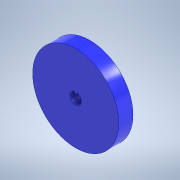
# Autodesk Inventor part: celestronMountDecHandle
Saved by Autodesk Inventor 2021.1 (Build 251245000, 245)
## iProperties
Created: 2020-07-29
Part Number: celestronMountDecHandle
Material: PC/ABS Plastic
Document SubType Name: Modeling
Designer: robst
Density: 0.357273 g/cm^3
Appearance: Blue - Wall Paint - Glossy
Author: robst
Autodesk Inventor part; units mm, degrees
ref_plane "YZ Plane" through (0, 0, 0) normal (1, 0, 0) x (0, 1, 0)
ref_plane "XY Plane" through (0, 0, 0) normal (0, 0, 1) x (1, 0, 0)
sketch "Sketch1" plane through (0, 0, 0) normal (0, 0, 1) x (1, 0, 0)
  circle A0 centre (0, 0) radius 38.1
  dimension "d0" = 76.2
  constraints: 1 centre point, 1 coincident
  measures "d0" diameter of A0
extrude "Extrusion1" add sketch "Sketch1" against normal blind 12.7
sketch "Sketch2" plane through (0, 0, -12.7) normal (0, 0, -1) x (-1, 0, 0)
  circle A0 centre (0, 0) radius 15.1765
  dimension "d3" = 30.353
  constraints: 1 centre point, 1 coincident
  measures "d3" diameter of A0
extrude "Extrusion2" add sketch "Sketch2" along normal blind 12.7
sketch "Sketch3" plane through (0, 0, 0) normal (0, 0, 1) x (1, 0, 0)
  arc A0 (-1.1906, 4.8732) -> (1.1906, 4.8732) centre (0, 0) ccw
  line L0 (-1.1906, 4.8732) -> (-1.1906, 3.4285)
  line L1 (-1.1906, 3.4285) -> (1.1906, 3.4285)
  line L2 (1.1906, 3.4285) -> (1.1906, 4.8732)
  circle A1 centre (0, 0) radius 15.1765 projected
  dimension "d6" = 10.033
  dimension "d7" = 2.3813
  dimension "d8" = 1.4446
  dimension "d15" = 10.16
  constraints: 6 end point, 2 point on circle, 2 vertical, 1 centre point, 1 coincident, 1 horizontal, 1 parallel
  measures "d6" diameter of A0
  measures "d7" distance of L0.end L1.end
  measures "d8" distance of L0.start L0.end
  measures "d15" radial gap between concentric circles of A0 A1
extrude "Extrusion3" cut sketch "Sketch3" against normal through all contours L0 L1 L2 A0
ref_plane "Work Plane2" through (0, -15.1765, 0) normal (0, 1, 0) x (-1, 0, 0)
sketch "Sketch4" plane through (0, -15.1765, 0) normal (0, 1, 0) x (-1, 0, 0)
  line L0 (-15.1765, -12.7) -> (-15.1765, -25.4) projected
  line L1 (15.1765, -12.7) -> (15.1765, -25.4) projected
  line L2 (-38.1, -12.7) -> (38.1, -12.7) projected
  line L3 (-15.1765, -25.4) -> (15.1765, -25.4) projected
  line L4 (0, -25.4) -> (0, -12.7) construction
  point P0 (0, 0)
  point P1 (0, -19.05)
  constraints: 3 midpoint, 2 end point
hole "Hole1" at (0, -15.1765, -19.05) direction (0, 1, 0) diameter 5.1054 depth 11.43 counterbore diameter 6.5278 counterbore depth 7.874 clearance for "Hex Machine Screw" size "#10" standard "Ansi Unified Screw Threads"
sketch "Sketch5" plane through (0, 0, -12.7) normal (0, 0, -1) x (-1, 0, 0)
  circle A0 centre (0, 0) radius 25.4 construction
  line L0 (-28.0674, 5.9618) -> (-22.0201, 3.0404)
  line L1 (-22.0201, 3.0404) -> (-22.1276, 2.1359)
  line L2 (-22.1276, 2.1359) -> (-28.6914, 0.7139)
  line L3 (-28.6914, 0.7139) -> (-28.5844, 1.6133)
  line L4 (-28.5844, 1.6133) -> (-23.139, 2.7381)
  line L5 (-23.139, 2.7381) -> (-28.1689, 5.1084)
  line L6 (-28.1689, 5.1084) -> (-28.0674, 5.9618)
  spline S0 degree 2 poles (-23.232, 10.4675) (-21.6233, 9.8922) (-20.4509, 8.4181) (-20.7992, 7.4442) knots 0 0 0 1 2 2 2
  spline S1 degree 2 poles (-20.7992, 7.4442) (-21.1527, 6.4557) (-23.0196, 6.0796) (-24.5944, 6.6428) knots 0 0 0 1 2 2 2
  spline S2 degree 2 poles (-24.5944, 6.6428) (-26.2127, 7.2216) (-27.3754, 8.6922) (-27.0254, 9.6709) knots 0 0 0 1 2 2 2
  spline S3 degree 2 poles (-27.0254, 9.6709) (-26.6736, 10.6545) (-24.7921, 11.0255) (-23.232, 10.4675) knots 0 0 0 1 2 2 2
  spline S4 degree 2 poles (-21.7775, 8.7887) (-22.0315, 9.0107) (-22.9077, 9.4334) (-23.5231, 9.6535) knots 0 0 0 1 2 2 2
  spline S5 degree 2 poles (-23.5231, 9.6535) (-24.1384, 9.8735) (-25.0792, 10.1007) (-25.4277, 10.0887) knots 0 0 0 1 2 2 2
  spline S6 degree 2 poles (-25.4277, 10.0887) (-25.7763, 10.0768) (-26.242, 9.7679) (-26.3616, 9.4335) knots 0 0 0 1 2 2 2
  spline S7 degree 2 poles (-26.3616, 9.4335) (-26.4812, 9.0992) (-26.3204, 8.5553) (-26.0506, 8.3167) knots 0 0 0 1 2 2 2
  spline S8 degree 2 poles (-26.0506, 8.3167) (-25.7886, 8.0864) (-24.8895, 7.6665) (-24.3032, 7.4568) knots 0 0 0 1 2 2 2
  spline S9 degree 2 poles (-24.3032, 7.4568) (-23.6733, 7.2315) (-22.8025, 7.0075) (-22.428, 7.0157) knots 0 0 0 1 2 2 2
  spline S10 degree 2 poles (-22.428, 7.0157) (-22.0763, 7.0211) (-21.5878, 7.3327) (-21.463, 7.6816) knots 0 0 0 1 2 2 2
  spline S11 degree 2 poles (-21.463, 7.6816) (-21.3451, 8.0111) (-21.5059, 8.5549) (-21.7775, 8.7887) knots 0 0 0 1 2 2 2
  line L7 (-17.8094, 13.4448) -> (-19.8797, 10.1209)
  line L8 (-19.8797, 10.1209) -> (-20.6441, 10.597)
  spline S12 degree 2 poles (-20.6441, 10.597) (-20.7573, 11.1646) (-20.9847, 12.1914) (-21.1306, 12.7066) knots 0 0 0 1 2 2 2
  spline S13 degree 2 poles (-21.1306, 12.7066) (-21.4241, 13.7442) (-21.9563, 14.7001) (-22.3887, 14.9694) knots 0 0 0 1 2 2 2
  spline S14 degree 2 poles (-22.3887, 14.9694) (-22.6158, 15.1109) (-23.0436, 15.1833) (-23.2317, 15.1247) knots 0 0 0 1 2 2 2
  spline S15 degree 2 poles (-23.2317, 15.1247) (-23.4198, 15.066) (-23.7357, 14.8021) (-23.8609, 14.6011) knots 0 0 0 1 2 2 2
  spline S16 degree 2 poles (-23.8609, 14.6011) (-23.9806, 14.4089) (-24.1293, 13.956) (-24.1666, 13.7307) knots 0 0 0 1 2 2 2
  spline S17 degree 2 poles (-24.1666, 13.7307) (-24.2007, 13.5397) (-24.2028, 13.147) (-24.1961, 13.0215) knots 0 0 0 1 2 2 2
  line L9 (-24.1961, 13.0215) -> (-24.2205, 12.9822)
  line L10 (-24.2205, 12.9822) -> (-24.9893, 13.461)
  spline S18 degree 2 poles (-24.9893, 13.461) (-24.9597, 13.7518) (-24.6759, 14.6844) (-24.4528, 15.0426) knots 0 0 0 1 2 2 2
  spline S19 degree 2 poles (-24.4528, 15.0426) (-23.9822, 15.7982) (-22.6523, 16.1521) (-21.9709, 15.7277) knots 0 0 0 1 2 2 2
  spline S20 degree 2 poles (-21.9709, 15.7277) (-21.6521, 15.5291) (-21.2117, 15.0487) (-21.0662, 14.7762) knots 0 0 0 1 2 2 2
  spline S21 degree 2 poles (-21.0662, 14.7762) (-20.9119, 14.4982) (-20.6856, 13.8299) (-20.5935, 13.4814) knots 0 0 0 1 2 2 2
  spline S22 degree 2 poles (-20.5935, 13.4814) (-20.4344, 12.9095) (-20.1591, 11.5801) (-20.0826, 11.1869) knots 0 0 0 1 2 2 2
  line L11 (-20.0826, 11.1869) -> (-18.434, 13.8339)
  line L12 (-18.434, 13.8339) -> (-17.8094, 13.4448)
  dimension "d24" = 50.8
  constraints: 1 centre point, 1 coincident, 1 other
  measures "d24" diameter of A0
extrude "Extrusion4" cut sketch "Sketch5" against normal blind 2.54
equation "\"d0\" = outerDiameter"
equation "\"d1\" = handleThickness"
equation "\"d3\" = shaftOutsideDiameter"
equation "\"d4\" = shaftLength"
equation "\"d6\" = shaftDiameter"
equation "\"d7\" = keyWidth"
equation "\"d8\" = keyDepth"
equation "\"outerDiameter\" = 76.2"
equation "\"handleThickness\" = 12.7"
equation "\"totalLength\" = 25.4"
equation "\"shaftDiameter\" = 10.033"
equation "\"keyWidth\" = 2.38125"
equation "\"keyDepth\" = 1.44462"
equation "\"shaftLength\" = totalLength - handleThickness"
equation "\"shaftOutsideDiameter\" = shaftDiameter + 2 * setScrewDepth"
equation "\"setScrewDepth\" = 10.16"
equation "\"setScrewWorkPlane\" = 0.5 * shaftOutsideDiameter"
equation "\"d16\" = -setScrewWorkPlane"
body "Solid1"
